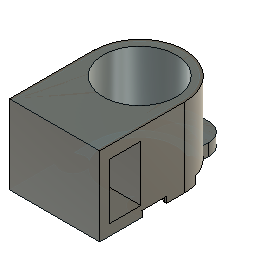
Motor hosing V6 (Autodesk Fusion 360 design; units mm, degrees)
Autodesk Fusion 360 part; units mm, degrees
sketch "Sketch1" plane through (0, 0, 0) normal (0, 0, 1) x (1, 0, 0)
  circle A0 centre (0, 0) radius 30
  dimension "d1" = 60
  constraint coincident A0.centre origin
  measures "d1" diameter of A0
sketch "Sketch2" plane through (0, 0, 0) normal (0, 0, 1) x (1, 0, 0)
  circle A0 centre (0, 0) radius 35.0151
  circle A1 centre (0, 0) radius 37.5
  dimension "d16" = 75
  constraint coincident A0.centre A1.centre
  measures "d16" diameter of A1
extrude "Extrude1" add sketch "Sketch2" along normal blind 65 contours A0
extrude "Extrude2" cut sketch "Sketch1" along normal blind 65
sketch "Sketch3" plane through (0, 0, 0) normal (0, 0, 1) x (1, 0, 0)
sketch "Sketch5" plane through (0, 0, 65) normal (0, 0, 1) x (-1, 0, 0)
sketch "Sketch7" plane through (0, 0, 65) normal (0, 0, 1) x (1, 0, 0)
sketch "Sketch8" plane through (0, 0, 65) normal (0, 0, 1) x (-1, 0, 0)
  circle A0 centre (0, 0) radius 30
  circle A1 centre (0, 0) radius 35.0151
  line L0 (-35.0151, 0) -> (35.3466, 0)
  line L1 (35.3466, 0) -> (35.3466, 70)
  line L2 (35.3466, 70) -> (-35.0151, 70)
  line L3 (-35.0151, 70) -> (-35.0151, 0)
  dimension "d7" = 70
  constraint horizontal L0
  constraint vertical L1
  constraint horizontal L2
  constraint vertical L3
  constraint coincident A1 L0.start
  measures "d7" distance of L0.start L2.end
extrude "Extrude3" add sketch "Sketch8" against normal blind 65 contours A1 L0 L1 L2 L3
sketch "Sketch9" plane through (-35.3466, 0, 0) normal (-1, 0, 0) x (0, -1, 0)
  line L0 (70, 65) -> (0, 65)
  line L1 (0, 65) -> (0, 0)
  line L2 (0, 0) -> (70, 0)
  line L3 (70, 0) -> (70, 65)
  line L4 (62, 55) -> (36, 55)
  line L5 (36, 55) -> (36, 9)
  line L6 (36, 9) -> (62, 9)
  line L7 (62, 9) -> (62, 55)
  constraint horizontal L4
  constraint vertical L5
  constraint horizontal L6
  constraint vertical L7
extrude "Extrude4" cut sketch "Sketch9" against normal blind 89 contours L4 L5 L6 L7
sketch "Sketch10" plane through (0, 0, 0) normal (0, 0, -1) x (1, 0, 0)
  circle A0 centre (0, 0) radius 30
  arc A1 (-35.0151, 0) -> (35.0151, 0) centre (0, 0) ccw
  line L0 (35.0151, 0) -> (35.0151, 70)
  line L1 (35.0151, 70) -> (-35.3466, 70)
  line L2 (-35.3466, 70) -> (-35.3466, 0)
  line L3 (-35.3466, 0) -> (-35.0151, 0)
  circle A2 centre (-30, 25) radius 10.1729
  circle A3 centre (30, 25) radius 11.2817
extrude "Extrude5" cut sketch "Sketch10" against normal blind 5 contours A0 L0 A3 | A0 L2 A2
sketch "Sketch11" plane through (0, 0, 0) normal (0, 0, -1) x (1, 0, 0)
  arc A0 (26.361, 14.3213) -> (35.0151, 14.8942) centre (30, 25) ccw
  arc A1 (-25.4341, 15.9094) -> (26.361, 14.3213) centre (0, 0) ccw
  arc A2 (-35.3466, 16.3455) -> (-25.4341, 15.9094) centre (-30, 25) ccw
  line L0 (-35.3466, 16.3455) -> (-35.3466, 0)
  line L1 (-35.3466, 0) -> (-35.0151, 0)
  arc A3 (-35.0151, 0) -> (35.0151, 0) centre (0, 0) ccw
  line L2 (35.0151, 0) -> (35.0151, 14.8942)
  circle A4 centre (24.1576, -21.6057) radius 10.7407
extrude "Extrude6" cut sketch "Sketch11" against normal blind 5 contours A1 A3 A4
sketch "Sketch12" plane through (0, 0, 65) normal (0, 0, 1) x (-1, 0, 0)
  circle A0 centre (0, 0) radius 30
  arc A1 (-35.0151, 0) -> (35.0151, 0) centre (0, 0) ccw
  line L0 (35.0151, 0) -> (35.3466, 0)
  line L1 (35.3466, 0) -> (35.3466, 70)
  line L2 (35.3466, 70) -> (-35.0151, 70)
  line L3 (-35.0151, 70) -> (-35.0151, 0)
extrude "Extrude7" add 1 faces at (35.0151, -16.9647, 41.6667) along direction (1, 0, 0) blind 2
extrude "Extrude8" add 1 faces at (-35.3466, -17.4485, 41.6667) along direction (-1, 0, 0) blind 2
sketch "Sketch13" plane through (0, 0, 65) normal (0, 0, 1) x (-1, 0, 0)
  circle A0 centre (0, 0) radius 37
  dimension "d21" = 74
  constraint coincident A0.centre origin
  measures "d21" diameter of A0
extrude "Extrude9" add sketch "Sketch13" against normal blind 60
sketch "Sketch14" plane through (0, 0, 5) normal (0, 0, -1) x (1, 0, 0)
  arc A0 (14.4835, -26.2722) -> (17.7176, -30.2017) centre (24.1576, -21.6057) ccw
  arc A1 (-35.0151, 0) -> (17.7176, -30.2017) centre (0, 0) ccw
  line L0 (-35.0151, 0) -> (-37, 0)
  arc A2 (-37, 0) -> (37, 0) centre (0, 0) ccw
  line L1 (37, 0) -> (35.0151, 0)
  arc A3 (31.9843, -14.25) -> (35.0151, 0) centre (0, 0) ccw
  arc A4 (31.9843, -14.25) -> (27.7196, -11.4728) centre (24.1576, -21.6057) ccw
  arc A5 (27.7196, -11.4728) -> (26.361, 14.3213) centre (0, 0) ccw
  arc A6 (26.361, 14.3213) -> (35.0151, 14.8942) centre (30, 25) ccw
  line L2 (35.0151, 14.8942) -> (37.0151, 14.8942)
  line L3 (37.0151, 14.8942) -> (37.0151, 35.1058)
  line L4 (37.0151, 35.1058) -> (35.0151, 35.1058)
  arc A7 (35.0151, 35.1058) -> (18.8401, 23.3463) centre (30, 25) ccw
  arc A8 (18.8401, 23.3463) -> (-20.2351, 22.1482) centre (0, 0) ccw
  arc A9 (-20.2351, 22.1482) -> (-35.3466, 33.6545) centre (-30, 25) ccw
  line L5 (-35.3466, 33.6545) -> (-37.3466, 33.6545)
  line L6 (-37.3466, 33.6545) -> (-37.3466, 16.3455)
  line L7 (-37.3466, 16.3455) -> (-35.3466, 16.3455)
  arc A10 (-35.3466, 16.3455) -> (-25.4341, 15.9094) centre (-30, 25) ccw
  arc A11 (-25.4341, 15.9094) -> (14.4835, -26.2722) centre (0, 0) ccw
  circle A12 centre (0, 0) radius 30
  dimension "d24" = 60
  constraint concentric A1 A12
  measures "d24" diameter of A12
extrude "Extrude10" cut sketch "Sketch14" against normal blind 60 contours A5 A8 A11 A12
extrude "Extrude11" add 1 faces at (29.4932, 16.7299, 5) along direction (0, 0, -1) blind 5
sketch "Sketch15" plane through (0, 0, 0) normal (0, 0, -1) x (1, 0, 0)
  line L0 (37, 0) -> (37.0151, 0)
  line L1 (37.0151, 0) -> (37.0151, 14.8942)
  line L2 (37.0151, 14.8942) -> (35.0151, 14.8942)
  arc A0 (26.361, 14.3213) -> (35.0151, 14.8942) centre (30, 25) ccw
  arc A1 (-25.4341, 15.9094) -> (26.361, 14.3213) centre (0, 0) ccw
  arc A2 (-35.3466, 16.3455) -> (-25.4341, 15.9094) centre (-30, 25) ccw
  line L3 (-35.3466, 16.3455) -> (-37.3466, 16.3455)
  line L4 (-37.3466, 16.3455) -> (-37.3466, 0)
  line L5 (-37.3466, 0) -> (-37, 0)
  arc A3 (-37, 0) -> (37, 0) centre (0, 0) ccw
  circle A4 centre (25, -21) radius 14.7648
extrude "Extrude12" cut sketch "Sketch15" against normal blind 6 contours A1 A3 A4
sketch "Sketch16" plane through (0, 0, 0) normal (0, 0, -1) x (1, 0, 0)
  arc A0 (11.7863, -27.5877) -> (16.5371, -33.0987) centre (25, -21) ccw
  arc A1 (-25.4341, 15.9094) -> (11.7863, -27.5877) centre (0, 0) ccw
  arc A2 (-35.3466, 16.3455) -> (-25.4341, 15.9094) centre (-30, 25) ccw
  line L0 (-35.3466, 16.3455) -> (-37.3466, 16.3455)
  line L1 (-37.3466, 16.3455) -> (-37.3466, 0)
  line L2 (-37.3466, 0) -> (-37, 0)
  arc A3 (-37, 0) -> (16.5371, -33.0987) centre (0, 0) ccw
  line L3 (-20, -30) -> (22, -30)
  line L4 (22, -30) -> (22, -42)
  line L5 (22, -42) -> (-20, -42)
  line L6 (-20, -42) -> (-20, -30)
  constraint horizontal L3
  constraint vertical L4
  constraint horizontal L5
  constraint vertical L6
sketch "Sketch18" plane through (0, 0, 0) normal (0, 0, -1) x (1, 0, 0)
  arc A0 (11.7863, -27.5877) -> (16.5371, -33.0987) centre (25, -21) ccw
  arc A1 (-25.4341, 15.9094) -> (11.7863, -27.5877) centre (0, 0) ccw
  arc A2 (-35.3466, 16.3455) -> (-25.4341, 15.9094) centre (-30, 25) ccw
  line L0 (-35.3466, 16.3455) -> (-37.3466, 16.3455)
  line L1 (-37.3466, 16.3455) -> (-37.3466, 0)
  line L2 (-37.3466, 0) -> (-37, 0)
  arc A3 (-37, 0) -> (16.5371, -33.0987) centre (0, 0) ccw
sketch "Sketch19" plane through (0, 0, 0) normal (0, 0, -1) x (1, 0, 0)
  line L0 (-20, -30) -> (21, -30)
  line L1 (21, -30) -> (21, -42)
  line L2 (21, -42) -> (-20, -42)
  line L3 (-20, -42) -> (-20, -30)
  constraint horizontal L0
  constraint vertical L1
  constraint horizontal L2
  constraint vertical L3
extrude "Extrude14" add sketch "Sketch19" against normal blind 10
extrude "Extrude15" add 1 faces at (7.3333, 42, 6.6667) along direction (0, 1, 0) blind 5
extrude "Extrude16" add 1 faces at (7.3333, 47, 6.6667) along direction (0, 1, 0) blind 4
fillet "Fillet8" radius 15 1 edges at (-20, 51, 5)
fillet "Fillet9" radius 15 1 edges at (21, 51, 5)
hole "Hole2" at (-0.083, 42.7851, 10) direction (0, 0, -1) diameter 6.3 depth 15 tip angle 118
sketch "Sketch20" plane through (0, 0, 10) normal (0, 0, 1) x (-1, 0, 0)
  circle A0 centre (0.083, -42.7851) radius 3.15
  arc A1 (-21, -36) -> (-6, -51) centre (-6, -36) ccw
  line L0 (-6, -51) -> (5, -51)
  arc A2 (5, -51) -> (20, -36) centre (5, -36) ccw
  line L1 (20, -36) -> (20, -31.1288)
  arc A3 (-21, -30.4631) -> (20, -31.1288) centre (0, 0) ccw
  line L2 (-21, -30.4631) -> (-21, -36)
sketch "Sketch21" plane through (0, 0, 0) normal (0, 0, -1) x (1, 0, 0)
  arc A0 (35.0151, 35.1058) -> (18.8401, 23.3463) centre (30, 25) ccw
  line L0 (35.0151, 35.1058) -> (37.0151, 35.1058)
  line L1 (37.0151, 35.1058) -> (37.0151, 70)
  line L2 (37.0151, 70) -> (-37.3466, 70)
  line L3 (-37.3466, 70) -> (-37.3466, 33.6545)
  line L4 (-37.3466, 33.6545) -> (-35.3466, 33.6545)
  arc A1 (-20.2351, 22.1482) -> (-35.3466, 33.6545) centre (-30, 25) ccw
  arc A2 (18.8401, 23.3463) -> (-20.2351, 22.1482) centre (0, 0) ccw
hole "Hole3" at (10.0299, -50.0019, 0) direction (0, 0, 1) diameter 6.3 depth 15 tip angle 118
hole "Hole4" at (-9.9726, -50.1489, 0) direction (0, 0, 1) diameter 6.3 depth 15 tip angle 118
sketch "Sketch22" plane through (0, 0, 0) normal (0, 0, -1) x (1, 0, 0)
sketch "Sketch23" plane through (0, 0, 0) normal (0, 0, 1) x (1, 0, 0)
sketch "Sketch24" plane through (0, 0, 0) normal (0, 0, -1) x (1, 0, 0)
  circle A0 centre (-0.083, -42.7851) radius 3.15
  arc A1 (6, -51) -> (21, -36) centre (6, -36) ccw
  line L0 (21, -36) -> (21, -30)
  line L1 (21, -30) -> (13.2953, -30)
  arc A2 (11.7863, -27.5877) -> (13.2953, -30) centre (25, -21) ccw
  arc A3 (-25.4341, 15.9094) -> (11.7863, -27.5877) centre (0, 0) ccw
  arc A4 (-35.3466, 16.3455) -> (-25.4341, 15.9094) centre (-30, 25) ccw
  line L2 (-35.3466, 16.3455) -> (-37.3466, 16.3455)
  line L3 (-37.3466, 16.3455) -> (-37.3466, 0)
  line L4 (-37.3466, 0) -> (-37, 0)
  arc A5 (-37, 0) -> (-20, -31.1288) centre (0, 0) ccw
  line L5 (-20, -31.1288) -> (-20, -36)
  arc A6 (-20, -36) -> (-5, -51) centre (-5, -36) ccw
  line L6 (-5, -51) -> (6, -51)
